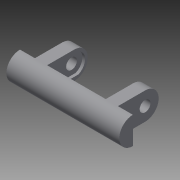
# Autodesk Inventor part: Sliide
Saved by Autodesk Inventor 2014 SP1 (Build 180222100, 222)
## iProperties
Created: 2016-12-01
Part Number: Sliide
Material: Generic
Document SubType Name: Modeling
Designer: danielsikar
Density: 1 g/cm^3
Appearance: Default
Author: danielsikar
Autodesk Inventor part; units mm, degrees
ref_plane "YZ Plane" through (0, 0, 0) normal (1, 0, 0) x (0, 1, 0)
ref_plane "XZ Plane" through (0, 0, 0) normal (0, 1, 0) x (-1, 0, 0)
ref_plane "XY Plane" through (0, 0, 0) normal (0, 0, 1) x (1, 0, 0)
sketch "Sketch1" plane through (0, 0, 0) normal (0, 0, 1) x (1, 0, 0)
  line L0 (0, 0) -> (41.6, 0)
  line L1 (41.6, 0) -> (41.6, 20)
  line L2 (41.6, 20) -> (0, 20)
  line L3 (0, 20) -> (0, 0)
  dimension "d0" = 41.6
  dimension "d1" = 20
  constraints: 8 end point, 2 parallel, 1 horizontal, 1 perpendicular
  measures "d0" distance of L2.end L1.end
  measures "d1" distance of L1.end L0.end
extrude "Extrusion1" add sketch "Sketch1" along normal blind 10
sketch "Sketch3" plane through (0, 0, 10) normal (0, 0, 1) x (1, 0, 0)
  line L0 (0, 20) -> (5, 20)
  line L1 (5, 20) -> (5, 10)
  line L2 (5, 10) -> (0, 10)
  line L3 (0, 10) -> (0, 20)
  line L4 (41.6, 20) -> (36.6, 20)
  line L5 (36.6, 20) -> (36.6, 10)
  line L6 (36.6, 10) -> (41.6, 10)
  line L7 (41.6, 10) -> (41.6, 20)
  dimension "d7" = 5
  dimension "d8" = 5
  dimension "d9" = 10
  constraints: 16 end point, 4 parallel, 2 horizontal, 2 perpendicular
  measures "d7" distance of L1.end L2.end
  measures "d8" distance of L6.end L5.end
  measures "d9" distance of L5.end L4.end
extrude "Extrusion2" cut sketch "Sketch3" against normal through all
sketch "Sketch4" plane through (0, 0, 10) normal (0, 0, 1) x (1, 0, 0)
  line L0 (36.6, 20) -> (5, 20) projected
  line L1 (5, 20) -> (5, 10) projected
  line L2 (10, 20) -> (31.6, 20)
  line L3 (31.6, 20) -> (31.6, 10)
  line L4 (31.6, 10) -> (10, 10)
  line L5 (10, 10) -> (10, 20)
  dimension "d12" = 21.6
  dimension "d13" = 10
  dimension "d14" = 5
  constraints: 8 end point, 2 parallel, 1 horizontal, 1 perpendicular, 1 point on line
  measures "d12" distance of L3.end L4.end
  measures "d13" distance of L2.end L3.end
  measures "d14" distance between parallel lines of L1 L5
extrude "Extrusion3" cut sketch "Sketch4" against normal through all
fillet "Fillet1" radius 5 6 edges at (20.8, 0, 0) (20.8, 0, 10) (34.1, 20, 10) (34.1, 20, 0) (7.5, 20, 0) (7.5, 20, 10)
sketch "Sketch5" plane through (10, 10, 10) normal (0, 1, 0) x (1, 0, 0)
  line L0 (0, 10) -> (21.6, 10) projected
  line L1 (0, 0) -> (0, 10) projected
  line L2 (21.6, 0) -> (0, 0) projected
  line L3 (21.6, 0) -> (21.6, 10) projected
  point P0 (-10, 10)
extrude "Extrusion4" cut sketch "Sketch5" against normal blind 5
sketch "Sketch6" plane through (36.6, 10, 10) normal (0, 1, 0) x (1, 0, 0)
  line L0 (0, 10) -> (5, 10) projected
  line L1 (0, 0) -> (0, 10) projected
  line L2 (5, 0) -> (0, 0) projected
  line L3 (5, 10) -> (5, 0) projected
  point P0 (-36.6, 10)
extrude "Extrusion5" cut sketch "Sketch6" against normal blind 5
sketch "Sketch7" plane through (0, 10, 10) normal (0, 1, 0) x (1, 0, 0)
  line L0 (0, 10) -> (5, 10) projected
  line L1 (0, 0) -> (0, 10) projected
  line L2 (5, 0) -> (0, 0) projected
  line L3 (5, 0) -> (5, 10) projected
extrude "Extrusion6" cut sketch "Sketch7" against normal blind 5
sketch "Sketch8" plane through (5, 15, 5) normal (-1, 0, 0) x (0, 0, 1)
  arc A0 (5, 0) -> (-5, 0) centre (0, 0) ccw projected
  line L0 (-5, -10) -> (-5, 0) projected
  line L1 (-5, -10) -> (5, -10) projected
  line L2 (5, 0) -> (5, -10) projected
  point P0 (-5, -15)
extrude "Extrusion7" cut sketch "Sketch8" against normal blind 0.5
sketch "Sketch9" plane through (36.6, 15, 5) normal (1, 0, 0) x (0, 0, -1)
  arc A0 (5, 0) -> (-5, 0) centre (0, 0) ccw projected
  line L0 (-5, -10) -> (-5, 0) projected
  line L1 (-5, -10) -> (5, -10) projected
  line L2 (5, 0) -> (5, -10) projected
  point P0 (5, -15)
extrude "Extrusion8" cut sketch "Sketch9" against normal blind 0.5
sketch "Sketch10" plane through (36.1, 15, 5) normal (1, 0, 0) x (0, 0, -1)
  arc A0 (5, 0) -> (-5, 0) centre (0, 0) ccw projected
  circle A1 centre (0, 0) radius 2
  point P0 (5, -15)
  dimension "d28" = 4
  constraints: 1 centre point, 1 coincident
  measures "d28" diameter of A1
extrude "Extrusion9" cut sketch "Sketch10" against normal through all
sketch "Sketch11" plane through (31.6, 15, 5) normal (-1, 0, 0) x (0, 0, 1)
  circle A0 centre (0, 0) radius 2 projected
  arc A1 (5, 0) -> (-5, 0) centre (0, 0) ccw projected
  line L0 (5, 0) -> (5, -10) projected
  line L1 (-3.7, 1.5199) -> (-3.7, -1.5199)
  line L2 (3.7, 1.5199) -> (3.7, -1.5199)
  arc A2 (-3.7, -1.5199) -> (3.7, -1.5199) centre (0, 0) ccw
  arc A3 (3.7, 1.5199) -> (-3.7, 1.5199) centre (0, 0) ccw
  point P0 (-5, -15)
  dimension "d33" = 3.7
  constraints: 4 end point, 4 point on circle, 2 centre point, 2 parallel, 1 coincident
  measures "d33" distance from line of L1 A0.centre
extrude "Extrusion10" cut sketch "Sketch11" against normal blind 1
sketch "Sketch12" plane through (10, 15, 5) normal (1, 0, 0) x (0, 0, -1)
  circle A0 centre (0, 0) radius 2 projected
  arc A1 (5, 0) -> (-5, 0) centre (0, 0) ccw projected
  line L0 (5, 0) -> (5, -10) projected
  line L1 (3.7, 1.5199) -> (3.7, -1.5199)
  line L2 (-3.7, 1.5199) -> (-3.7, -1.5199)
  arc A2 (-3.7, -1.5199) -> (3.7, -1.5199) centre (0, 0) ccw
  arc A3 (3.7, 1.5199) -> (-3.7, 1.5199) centre (0, 0) ccw
  point P0 (5, -15)
  dimension "d37" = 3.7
  constraints: 4 end point, 4 point on circle, 2 centre point, 2 parallel, 1 coincident
  measures "d37" distance from line of L1 A2.centre
extrude "Extrusion11" cut sketch "Sketch12" against normal blind 1
body "Solid1"
